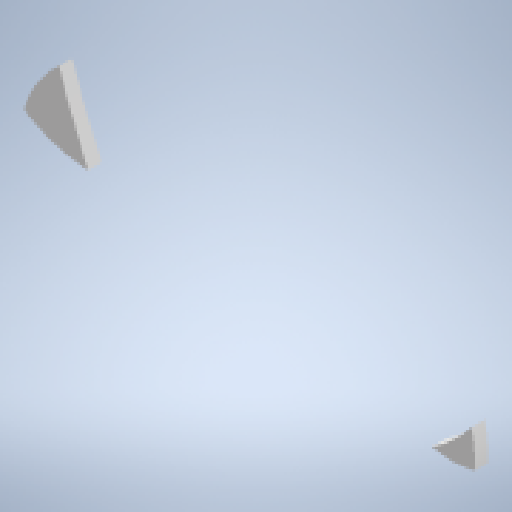
# Autodesk Inventor part: EarsPeach
Saved by Autodesk Inventor 2023 (Build 270158000, 158)
## iProperties
Created: 2022-11-09
Part Number: EarsPeach
Material: Generic
Document SubType Name: Modeling
Designer: reide
Density: 1 g/cm^3
Appearance: Default
Author: reide
Autodesk Inventor part; units mm, degrees
ref_plane "YZ Plane" through (0, 0, 0) normal (1, 0, 0) x (0, 1, 0)
ref_plane "XZ Plane" through (0, 0, 0) normal (0, 1, 0) x (-1, 0, 0)
ref_plane "XY Plane" through (0, 0, 0) normal (0, 0, 1) x (1, 0, 0)
sketch "Sketch1" plane through (0, 0, 0) normal (0, 0, 1) x (1, 0, 0)
  arc A0 (-5.2404, 49.7595) -> (-9.4372, 45.8783) centre (-4.3358, 44.5716) ccw projected
  ellipse E0 centre (-14.2006, 46.3092) end of major axis (-18.9639, 46.7402) minor radius 4.1297 (-9.5634, 45.2073) -> (-9.4372, 45.8783) ccw projected
  arc A1 (-9.4372, 45.8783) -> (-9.5634, 45.2073) centre (-4.3358, 44.5716) ccw projected
  ellipse E1 centre (-14.2006, 46.3092) end of major axis (-9.4372, 45.8783) minor radius 4.1297 (-9.4372, 45.8783) -> (-11.6728, 49.7595) ccw projected
  line L0 (-5.2404, 49.7595) -> (-11.6728, 49.7595) projected
  arc A2 (-63.9112, 49.7595) -> (-65.2479, 47.7205) centre (-46.6268, 36.9707) ccw projected
  spline S0 degree 3 poles (-61.2334, 46.0013) (-61.241, 45.9723) (-61.249, 45.9435) (-61.3795, 45.4969) (-61.5834, 45.1031) (-62.0656, 44.493) (-62.3191, 44.2564) (-62.8632, 43.9012) (-63.1479, 43.7731) (-63.7035, 43.6437) (-63.9708, 43.6275) (-64.3938, 43.6897) (-64.5534, 43.735) (-64.7038, 43.8014) (-64.988, 43.927) (-65.2364, 44.13) (-65.528, 44.5193) (-65.6143, 44.674) (-65.8392, 45.2168) (-65.8922, 45.6367) (-65.8223, 46.5736) (-65.6475, 47.0876) (-65.3313, 47.5991) (-65.2906, 47.6605) (-65.2479, 47.7205) knots -2.04297 -2.04297 -2.04297 -2.04297 -2.033998 -2.033998 -1.903383 -1.903383 -1.8007 -1.8007 -1.70847 -1.70847 -1.629539 -1.629539 -1.580207 -1.580207 -1.580207 -1.486994 -1.486994 -1.434286 -1.434286 -1.31073 -1.31073 -1.152429 -1.152429 -1.130329 -1.130329 -1.130329 -1.130329 projected
  arc A3 (-58.3708, 49.7595) -> (-61.2334, 46.0013) centre (-53.4946, 43.0761) ccw projected
  line L1 (-53.1262, 49.7595) -> (-58.3708, 49.7595) projected
  arc A4 (-53.1262, 49.7595) -> (-48.6958, 45.9623) centre (-39.6934, 60.9493) ccw projected
  arc A5 (-48.6958, 45.9623) -> (-57.6528, 37.9355) centre (-45.2762, 33.1357) ccw projected
  arc A6 (-57.6528, 37.9355) -> (-59.4928, 20.8874) centre (-29.8304, 26.3092) ccw projected
  arc A7 (-59.4928, 20.8874) -> (-66.5058, 9.6449) centre (-48.4804, 6.2092) ccw projected
  arc A8 (-66.5058, 9.6449) -> (-53.176, 5.3746) centre (-55.5804, 20.8092) ccw projected
  arc A9 (-53.176, 5.3746) -> (-7.6044, -3.2884) centre (-25.0596, 29.0848) ccw projected
  arc A10 (-7.6044, -3.2884) -> (5.496, -3.9781) centre (-0.2547, 11.5527) ccw projected
  arc A11 (5.496, -3.9781) -> (2.6997, 6.1416) centre (-9.1212, -2.5709) ccw projected
  arc A12 (2.6997, 6.1416) -> (5.3748, 19.6874) centre (-16.5082, 16.972) ccw projected
  arc A13 (5.3748, 19.6874) -> (-1.1492, 41.7351) centre (-4.3358, 28.8031) ccw projected
  arc A14 (-1.1492, 41.7351) -> (-3.5223, 48.7595) centre (-4.3358, 44.5716) ccw projected
  line L2 (-3.5223, 48.7595) -> (-2.143, 48.7595) projected
  arc A15 (-1.143, 49.7595) -> (-2.143, 48.7595) centre (-1.143, 48.7595) ccw projected
  line L3 (66.0202, 49.7595) -> (-1.143, 49.7595) projected
  line L4 (66.0202, 57.7611) -> (66.0202, 49.7595) projected
  line L5 (-65.756, 57.7611) -> (66.0202, 57.7611) projected
  arc A16 (-67.756, 59.7611) -> (-65.756, 57.7611) centre (-65.756, 59.7611) ccw projected
  line L6 (-67.756, 152.7595) -> (-67.756, 59.7611) projected
  arc A17 (-65.756, 154.7595) -> (-67.756, 152.7595) centre (-65.756, 152.7595) ccw projected
  line L7 (66.0202, 154.7595) -> (-65.756, 154.7595) projected
  line L8 (66.0202, 162.7595) -> (66.0202, 154.7595) projected
  line L9 (-71.181, 162.7595) -> (66.0202, 162.7595) projected
  arc A18 (-71.181, 162.7595) -> (-75.181, 158.7595) centre (-71.181, 158.7595) ccw projected
  line L10 (-75.181, 53.7595) -> (-75.181, 158.7595) projected
  arc A19 (-75.181, 53.7595) -> (-71.181, 49.7595) centre (-71.181, 53.7595) ccw projected
  line L11 (-63.9112, 49.7595) -> (-71.181, 49.7595) projected
  ellipse E2 centre (-14.9945, 46.3092) end of major axis (-19.4324, 46.3092) minor radius 3.9921 projected
  ellipse E3 centre (-31.5804, 27.2595) end of major axis (-34.5804, 27.2595) minor radius 2.4928 projected
  arc A20 (-58.7621, 19.1111) -> (-54.151, 7.251) centre (81.3354, 66.754) ccw projected
  arc A21 (-64.2817, 10.4994) -> (-54.151, 7.251) centre (-53.6108, 26.3569) ccw projected
  arc A22 (-58.7621, 19.1111) -> (-64.2817, 10.4994) centre (-45.7447, 4.6929) ccw projected
  arc A23 (-9.9763, 24.2915) -> (-11.5804, 23.2595) centre (-10.2045, 22.8836) ccw projected
  arc A24 (-11.5804, 23.2595) -> (-13.5065, 25.2338) centre (-14.5804, 22.2595) ccw projected
  ellipse E4 centre (-11.7362, 25.2595) end of major axis (-11.7362, 34.2595) minor radius 1.7702 (-9.9763, 24.2915) -> (-13.5065, 25.2338) ccw projected
  circle A25 centre (-2.5804, 20.8092) radius 2.7388 projected
  circle A26 centre (-24.5804, 22.2595) radius 2.8284 projected
  arc A27 (-3.4029, -2.7392) -> (2.8892, 3.0642) centre (-17.7337, 19.1111) ccw projected
  arc A28 (3.3474, -2.6578) -> (2.8892, 3.0642) centre (-14.8462, -1.2352) ccw projected
  arc A29 (-3.4029, -2.7392) -> (3.3474, -2.6578) centre (-0.2141, 12.7425) ccw projected
  ellipse E5 centre (-4.3358, 44.8225) end of major axis (-0.3171, 44.5466) minor radius 3.5714 projected
  ellipse E6 centre (3.8758, 24.0009) end of major axis (1.3443, 24.0009) minor radius 2.1289 projected
  arc A30 (3.2472, -2.5779) -> (2.812, 2.858) centre (-14.0367, -1.2265) ccw
  arc A31 (-3.1656, -2.6553) -> (3.2472, -2.5779) centre (-0.1362, 12.0523) ccw
  arc A32 (-64.0582, 10.5748) -> (-54.4339, 7.4888) centre (-53.9208, 25.6394) ccw
  arc A33 (-58.8145, 18.7559) -> (-64.0582, 10.5748) centre (-46.448, 5.0586) ccw
  arc A34 (-58.8145, 18.7559) -> (-54.4339, 7.4888) centre (74.2781, 64.0166) ccw
  arc A35 (-3.1656, -2.6553) -> (2.812, 2.858) centre (-16.7798, 18.1025) ccw
  point P0 (0, 0)
  point P1 (1.3443, -1.0602)
  point P2 (-59.8101, 12.0074)
  constraints: 12 point on circle, 6 centre point, 6 other
extrude "Extrusion1" add sketch "Sketch1" along normal blind 2 contours A31 A35 A30 | A33 A34 A32
body "Solid1"
